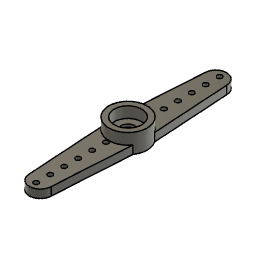
螺旋桨舵盘 v1 (Autodesk Fusion 360 design; units mm, degrees)
Autodesk Fusion 360 part; units mm, degrees
note: some values were not read from the file. Set by a fixed rule: which sketch regions a step uses.
sketch "草图1" plane through (0, 0, 0) normal (0, 1, 0) x (1, 0, 0)
  circle A0 centre (0, 0) radius 3.5
  line L0 (0, 0) -> (0, -16)
  line L1 (0, 0) -> (0, 16)
  circle A1 centre (0, -16) radius 2
  circle A2 centre (0, 16) radius 2
  line L2 (0, 16) -> (6, 16)
  line L3 (6, 16) -> (-7, 16)
  line L4 (2, 16) -> (2.8777, 2.0488)
  line L5 (2, 16) -> (15.9788, 16) construction
  line L6 (-2, 16) -> (-2.8733, 2.1192)
  line L7 (-2, 16) -> (11.9083, 16) construction
  line L8 (0, -16) -> (5, -16)
  line L9 (5, -16) -> (-6, -16)
  line L10 (2, -16) -> (2.8901, -1.8524)
  line L11 (2, -16) -> (16.1756, -16) construction
  line L12 (-2, -16) -> (-2.8817, -1.9865)
  line L13 (-2, -16) -> (12.0412, -16) construction
  line L14 (2.8777, 2.0488) -> (2.8885, 1.8784)
  line L15 (-2.8733, 2.1192) -> (-2.9, 1.6952)
  dimension "d1" = 7
  dimension "d2" = 16
  dimension "d3" = 16
  dimension "d4" = 4
  dimension "d5" = 4
  dimension "d6" = 86.4
  dimension "d7" = 93.6
  dimension "d8" = 13.9083
  dimension "d9" = 86.4
  dimension "d10" = 93.6
  constraint coincident A0.centre L0.start
  constraint vertical L0
  constraint parallel L0 L1
  constraint coincident L0.end A1.centre
  constraint coincident L1.end A2.centre
  constraint perpendicular L1 L2
  constraint perpendicular L1 L3
  constraint horizontal L5
  constraint coincident L2 L4.start
  constraint coincident A2 L4.start
  constraint horizontal L7
  constraint coincident A2 L6.start
  constraint coincident L3 L6.start
  constraint perpendicular L0 L8
  constraint perpendicular L0 L9
  constraint horizontal L11
  constraint coincident A1 L10.start
  constraint coincident L8 L10.start
  constraint horizontal L13
  constraint coincident A1 L12.start
  constraint coincident L9 L12.start
  constraint coincident A0 L12.end
  constraint parallel L4 L14
  constraint parallel L6 L15
  measures "d1" diameter of A0
  measures "d2" distance of A0.centre L0.end
  measures "d3" distance of A0.centre L1.end
  measures "d4" diameter of A1
  measures "d5" diameter of A2
  measures "d6" angle of L4 L5
  measures "d7" angle of L6 L7
  measures "d8" distance of L6.start L6.end
  measures "d9" angle of L10 L11
  measures "d10" angle of L12 L13
extrude "拉伸1" add sketch "草图1" along normal blind 1.5
sketch "草图2" plane through (0, 1.5, 0) normal (0, 1, 0) x (-1, 0, 0)
  arc A0 (-2, -16) -> (2, -16) centre (0, -16) ccw
  line L0 (2, -16) -> (2.8817, -1.9865)
  arc A1 (2.8817, -1.9865) -> (2.8817, 1.9865) centre (0, 0) ccw
  line L1 (2.8817, 1.9865) -> (2, 16)
  arc A2 (2, 16) -> (-2, 16) centre (0, 16) ccw
  line L2 (-2, 16) -> (-2.8817, 1.9865)
  arc A3 (-2.8817, 1.9865) -> (-2.8817, -1.9865) centre (0, 0) ccw
  line L3 (-2.8817, -1.9865) -> (-2, -16)
  circle A4 centre (0, 0) radius 3.5
  constraint coincident A1.centre A3.centre
extrude "拉伸2" add sketch "草图2" along normal blind 2 contours A1 A3 A4
sketch "草图3" plane through (0, 1.5, 0) normal (0, 1, 0) x (-1, 0, 0)
  arc A0 (-2.8817, -1.9865) -> (2.8817, -1.9865) centre (0, 0) ccw
  line L0 (-2.8817, -1.9865) -> (-2, -16)
  arc A1 (-2, -16) -> (2, -16) centre (0, -16) ccw
  line L1 (2, -16) -> (2.8817, -1.9865)
  line L2 (0, -4) -> (0, -16.75)
  line L3 (0, -16.75) -> (0, -14.2)
  line L4 (0, -14.2) -> (0, -11.65)
  line L5 (0, -11.65) -> (0, -9.1)
  line L6 (0, -9.1) -> (0, -6.55)
  circle A2 centre (0, -4) radius 0.45
  circle A3 centre (0, -16.75) radius 0.45
  circle A4 centre (0, -14.2) radius 0.45
  circle A5 centre (0, -11.65) radius 0.45
  circle A6 centre (0, -9.1) radius 0.45
  circle A7 centre (0, -6.55) radius 0.45
  line L7 (-8.6176, 0) -> (8, 0)
  circle A8 centre (0, 16.75) radius 0.45
  circle A9 centre (0, 14.2) radius 0.45
  circle A10 centre (0, 11.65) radius 0.45
  circle A11 centre (0, 9.1) radius 0.45
  circle A12 centre (0, 6.55) radius 0.45
  circle A13 centre (0, 4) radius 0.45
  dimension "d26" = 12.75
  dimension "d28" = 2.55
  dimension "d29" = 2.55
  dimension "d30" = 2.55
  dimension "d31" = 2.55
  dimension "d32" = 0.9
  dimension "d33" = 0.9
  dimension "d34" = 0.9
  dimension "d35" = 0.9
  dimension "d36" = 0.9
  dimension "d37" = 0.9
  constraint parallel L2 L3
  constraint parallel L2 L4
  constraint parallel L2 L5
  constraint parallel L2 L6
  constraint coincident L2.start A2.centre
  constraint coincident L2.end L3.start
  constraint coincident L3.end L4.start
  constraint coincident L4.end L5.start
  constraint coincident L5.end L6.start
  constraint coincident L6.end A7.centre
  constraint horizontal L7
  constraint symmetric A2 L7 A13
  constraint symmetric A3 L7 A8
  constraint symmetric A4 L7 A9
  constraint symmetric A5 L7 A10
  constraint symmetric A6 L7 A11
  constraint symmetric A7 L7 A12
  measures "d26" distance of L2.start L2.end
  measures "d28" distance of L2.end L3.end
  measures "d29" distance of L3.end L4.end
  measures "d30" distance of L4.end L5.end
  measures "d31" distance of L5.end L6.end
  measures "d32" diameter of A2
  measures "d33" diameter of A3
  measures "d34" diameter of A4
  measures "d35" diameter of A5
  measures "d36" diameter of A6
  measures "d37" diameter of A7
extrude "拉伸3" cut sketch "草图3" against normal blind 8 contours L2 L6 A7 | L2 L6 A7 | L2 L5 L6 A6 | L2 L5 L6 A6 | L2 L4 L5 A5 | L2 L4 L5 A5 | L2 L3 L4 A4 | L2 L3 L4 A4 | A2 | A3 | A8 | A9 | A10 | A11 | A12 | A13
sketch "草图4" plane through (0, 0, 0) normal (0, -1, 0) x (1, 0, 0)
  circle A0 centre (0, 11.65) radius 0.45
  circle A1 centre (0, -4) radius 0.45
  circle A2 centre (0, -14.2) radius 0.45
  circle A3 centre (0, -11.65) radius 0.45
  circle A4 centre (0, 4) radius 0.45
  circle A5 centre (0, 14.2) radius 0.45
  circle A6 centre (0, 9.1) radius 0.45
  circle A7 centre (0, -6.55) radius 0.45
  circle A8 centre (0, -16.75) radius 0.45
  circle A9 centre (0, -9.1) radius 0.45
  circle A10 centre (0, 6.55) radius 0.45
  circle A11 centre (0, 16.75) radius 0.45
  arc A12 (-2, -16) -> (2, -16) centre (0, -16) ccw
  line L0 (2, -16) -> (2.8817, -1.9865)
  arc A13 (2.8817, -1.9865) -> (2.8817, 1.9865) centre (0, 0) ccw
  line L1 (2.8817, 1.9865) -> (2, 16)
  arc A14 (2, 16) -> (-2, 16) centre (0, 16) ccw
  line L2 (-2, 16) -> (-2.8817, 1.9865)
  arc A15 (-2.8817, 1.9865) -> (-2.8817, -1.9865) centre (0, 0) ccw
  line L3 (-2.8817, -1.9865) -> (-2, -16)
  circle A16 centre (0, 0) radius 2.3
  dimension "d40" = 4.6
  constraint concentric A13 A16
  measures "d40" diameter of A16
extrude "拉伸4" cut sketch "草图4" against normal blind 1 contours A16
sketch "草图5" plane through (0, 1, 0) normal (0, -1, 0) x (1, 0, 0)
  circle A0 centre (0, 0) radius 2.3
  circle A1 centre (0, 0) radius 1.25
  dimension "d43" = 2.5
  constraint concentric A0 A1
  measures "d43" diameter of A1
extrude "拉伸5" cut sketch "草图5" against normal blind 10 contours A1
sketch "草图6" plane through (0, 3.5, 0) normal (0, 1, 0) x (-1, 0, 0)
  circle A0 centre (0, 0) radius 1.25
  circle A1 centre (0, 0) radius 3.5
  circle A2 centre (0, 0) radius 2.5
  dimension "d46" = 5
  constraint coincident A0.centre A1.centre
  measures "d46" diameter of A2
extrude "拉伸6" cut sketch "草图6" against normal blind 2 contours A2
